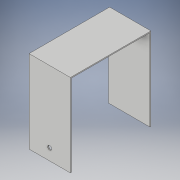
# Autodesk Inventor part: MAN_BASIS_SECONDARY_STRUCTURE
Saved by Autodesk Inventor 2019 (Build 230136000, 136)
## iProperties
Created: 2021-03-21
Part Number: MAN_BASIS_SECONDARY_STRUCTURE
Material: Generic
Document SubType Name: Modeling
Designer: DOMEK
Density: 1 g/cm^3
Appearance: Default
Author: DOMEK
Autodesk Inventor part; units mm, degrees
ref_plane "YZ Plane" through (0, 0, 0) normal (1, 0, 0) x (0, 1, 0)
ref_plane "XZ Plane" through (0, 0, 0) normal (0, 1, 0) x (-1, 0, 0)
ref_plane "XY Plane" through (0, 0, 0) normal (0, 0, 1) x (1, 0, 0)
sketch "Sketch2" plane through (0, 0, 0) normal (1, 0, 0) x (0, 1, 0)
  line L0 (0, 0) -> (80, 0)
  line L1 (80, 0) -> (80, 78)
  line L2 (80, 78) -> (0, 78)
  line L3 (0, 78) -> (0, 0)
  dimension "d3" = 80
  dimension "d4" = 78
  constraints: 8 end point, 2 parallel, 1 horizontal, 1 perpendicular
  measures "d3" distance of L2.end L1.end
  measures "d4" distance of L1.end L0.end
extrude "Extrusion2" add sketch "Sketch2" along normal blind 40
shell "Shell1" thickness 1 removed faces 3 at (13.3333, 0, 52) at (0, 26.6667, 52) at (40, 26.6667, 52)
sketch "Sketch3" plane through (0, 0, 78) normal (0, 0, 1) x (1, 0, 0)
  line L0 (0, 0) -> (40, 0) projected
  line L1 (0, 80) -> (40, 80) projected
  circle A0 centre (20, 11.1124) radius 2
  dimension "d8" = 4
  constraints: 1 centre point
  measures "d8" diameter of A0
extrude "Extrusion3" cut sketch "Sketch3" against normal blind 1
body "Solid2"
